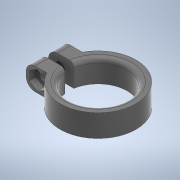
# Autodesk Inventor part: BallLock
Saved by Autodesk Inventor 2020.2 (Build 242310000, 310)
## iProperties
Created: 2021-06-30
Part Number: BallLock
Material: Generic
Document SubType Name: Modeling
Designer: JK
Density: 1 g/cm^3
Appearance: Smooth - Black
Author: JK
Autodesk Inventor part; units mm, degrees
ref_plane "YZ Plane" through (0, 0, 0) normal (1, 0, 0) x (0, 1, 0)
ref_plane "XZ Plane" through (0, 0, 0) normal (0, 1, 0) x (-1, 0, 0)
ref_plane "XY Plane" through (0, 0, 0) normal (0, 0, 1) x (1, 0, 0)
sketch "Sketch1" plane through (0, 0, 0) normal (0, 1, 0) x (-1, 0, 0)
  circle A0 centre (0, 0) radius 17
  circle A1 centre (0, 0) radius 13
  dimension "d0" = 26
  dimension "d1" = 34
  constraints: 2 centre point, 2 coincident
  measures "d0" diameter of A1
  measures "d1" diameter of A0
extrude "Extrusion1" add sketch "Sketch1" along normal blind 10
sketch "Sketch2" plane through (0, 10, 0) normal (0, 1, 0) x (1, 0, 0)
  line L0 (-21.6238, -8) -> (-8.7582, -8)
  line L1 (-8.7582, -8) -> (-8.7582, 8)
  line L2 (-8.7582, 8) -> (-21.6238, 8)
  line L3 (-21.6238, 8) -> (-21.6238, -8)
  point P0 (0, 0)
  dimension "d4" = 8
  dimension "d5" = 8
  constraints: 8 end point, 2 parallel, 1 horizontal, 1 perpendicular
  measures "d4" distance from line of L0 point (0, 0)
  measures "d5" distance from line of point (0, 0) L2
extrude "Extrusion2" cut sketch "Sketch2" against normal through all
sketch "Sketch3" plane through (0, 10, 0) normal (0, 1, 0) x (1, 0, 0)
  arc A0 (-10.247, -8) -> (-10.247, 8) centre (0, 0) ccw projected
  line L0 (-10.247, -8) -> (-24.247, -8)
  line L1 (-24.247, -8) -> (-24.247, -2)
  line L2 (-24.247, -2) -> (-10.247, -2)
  line L3 (-10.247, -2) -> (-10.247, -8)
  line L4 (-10.247, 8) -> (-24.247, 8)
  line L5 (-24.247, 8) -> (-24.247, 2)
  line L6 (-24.247, 2) -> (-10.247, 2)
  line L7 (-10.247, 2) -> (-10.247, 8)
  circle A1 centre (0, 0) radius 13
  point P0 (-10.247, -8)
  point P1 (-12.8452, -2)
  point P2 (-12.8452, 2)
  point P3 (-10.247, 8)
  dimension "d8" = 6
  dimension "d9" = 6
  dimension "d10" = 14
  constraints: 16 end point, 4 parallel, 2 horizontal, 2 perpendicular, 1 centre point, 1 coincident, 1 concentric, 1 point on line
  measures "d8" distance of L0.end L1.end
  measures "d9" distance of L4.end L5.end
  measures "d10" distance between parallel lines of L5 L7
extrude "Extrusion3" add sketch "Sketch3" against normal blind 10 contours L0 L1 L2 A1 | A1 L6 L5 L4
sketch "Sketch4" plane through (-24.247, 10, 8) normal (0, 0, 1) x (1, 0, 0)
  circle A0 centre (5, -5) radius 2.2
  line L0 (0, 0) -> (0, -10) projected
  line L1 (9.247, -10) -> (0, -10) projected
  point P0 (24.247, -10)
  dimension "d13" = 4.4
  dimension "d14" = 5
  dimension "d15" = 5
  constraints: 1 centre point
  measures "d13" diameter of A0
  measures "d14" distance from line of L0 A0.centre
  measures "d15" distance from line of L1 A0.centre
extrude "Extrusion4" cut sketch "Sketch4" against normal through all
sketch "Sketch5" plane through (-24.247, 10, 8) normal (0, 0, 1) x (1, 0, 0)
  circle A0 centre (5, -5) radius 2.2 projected
  circle A1 centre (5, -5) radius 3.6
  line L0 (5, -9.1569) -> (1.4, -7.0785)
  line L1 (1.4, -7.0785) -> (1.4, -2.9215)
  line L2 (1.4, -2.9215) -> (5, -0.8431)
  line L3 (5, -0.8431) -> (8.6, -2.9215)
  line L4 (8.6, -2.9215) -> (8.6, -7.0785)
  line L5 (8.6, -7.0785) -> (5, -9.1569)
  point P0 (24.247, -10)
  dimension "d18" = 7.2
  constraints: 12 end point, 2 coincident, 1 centre point, 1 tangent, 1 vertical alignment, 13 other
  measures "d18" diameter of A1
extrude "Extrusion5" cut sketch "Sketch5" against normal blind 3 contours A0 | A1 | L4 L5 A1 | A1 L3 L4 | A1 L2 L3 | L5 L0 A1 | A1 L1 L2 | L0 L1 A1
fillet "Fillet2" radius 4 4 edges at (-24.247, 10, 5) (-24.247, 10, -5) (-24.247, 0, -5) (-24.247, 0, 5)
fillet "Fillet3" radius 2 3 edges at (-11.9295, 10, -5.166) (13, 10, 0) (-11.9295, 10, 5.166)
body "Solid1"
